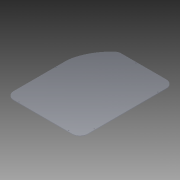
# Autodesk Inventor part: metacrilat proteccio dret
Saved by Autodesk Inventor 2012 SP1 (Build 160190100, 190)
## iProperties
Created: 2015-03-29
Part Number: metacrilat proteccio dret
Material: Default
Document SubType Name: Modeling
Designer: sheina
Density: 1 g/cm^3
Author: sheina
Autodesk Inventor part; units mm, degrees
ref_plane "YZ Plane" through (0, 0, 0) normal (1, 0, 0) x (0, 1, 0)
ref_plane "XZ Plane" through (0, 0, 0) normal (0, 1, 0) x (-1, 0, 0)
ref_plane "XY Plane" through (0, 0, 0) normal (0, 0, 1) x (1, 0, 0)
sketch "Boceto1" plane through (0, 0, 0) normal (0, 0, 1) x (1, 0, 0)
  line L0 (200.6138, -49.1011) -> (347.0892, -49.1011)
  line L1 (366.6054, -71.1) -> (366.6054, -332.1)
  line L2 (352.0892, -357.1011) -> (151.6064, -357.1011)
  line L3 (124.6054, -332.1) -> (124.6054, -152.9933)
  line L4 (366.6054, -332.1) -> (366.6054, -357.1011)
  line L5 (352.0892, -357.1011) -> (366.6054, -357.1011)
  line L6 (347.0892, -49.1011) -> (366.6054, -49.1011)
  line L7 (366.6054, -71.1) -> (366.6054, -49.1011)
  line L8 (151.6064, -357.1011) -> (124.6054, -357.1011)
  line L9 (124.6054, -332.1) -> (124.6054, -357.1011)
  line L10 (200.6138, -49.1011) -> (185.295, -49.1011)
  arc A0 (185.295, -49.1011) -> (124.6054, -152.9933) centre (292.3571, -181.3147) ccw
  dimension "d2" = 308
  dimension "d3" = 242
  constraints: 22 end point, 5 perpendicular, 2 parallel, 2 point on circle, 1 centre point
  measures "d2" distance between parallel lines of L2 L0
  measures "d3" distance between parallel lines of L3 L1
extrude "Extrusión2" add sketch "Boceto1" along normal blind 2
fillet "Empalme1" radius 25 3 edges at (366.6054, -49.1011, 1) (366.6054, -357.1011, 1) (124.6054, -357.1011, 1)
sketch "Boceto3" plane through (0, 0, 2) normal (0, 0, 1) x (1, 0, 0)
  line L0 (341.6054, -357.1011) -> (149.6054, -357.1011) projected
  line L1 (366.6054, -74.1011) -> (366.6054, -332.1011) projected
  line L2 (185.295, -49.1011) -> (341.6054, -49.1011) projected
  line L3 (124.6054, -332.1011) -> (124.6054, -152.9933) projected
  circle A0 centre (164.6054, -354.1011) radius 1.75
  circle A1 centre (326.6054, -354.1011) radius 1.75
  circle A2 centre (127.6054, -196.1011) radius 1.75
  circle A3 centre (363.6054, -307.1011) radius 1.75
  circle A4 centre (363.6054, -99.1011) radius 1.75
  circle A5 centre (245.1054, -52.1011) radius 1.75
  point P0 (200.6138, -49.1011)
  point P1 (0, 0)
  dimension "d7" = 3.5
  dimension "d8" = 3.5
  dimension "d9" = 3.5
  dimension "d10" = 3.5
  dimension "d11" = 3.5
  dimension "d12" = 3.5
  dimension "d13" = 3
  dimension "d14" = 3
  dimension "d15" = 3
  dimension "d16" = 3
  dimension "d17" = 3
  dimension "d18" = 3
  dimension "d19" = 121.5
  dimension "d20" = 161
  dimension "d21" = 50
  dimension "d22" = 50
  dimension "d23" = 40
  dimension "d24" = 40
  constraints: 6 centre point
  measures "d7" diameter of A0
  measures "d8" diameter of A1
  measures "d9" diameter of A2
  measures "d10" diameter of A3
  measures "d11" diameter of A4
  measures "d12" diameter of A5
  measures "d13" distance from line of L3 A2.centre
  measures "d14" distance from line of L0 A0.centre
  measures "d15" distance from line of L0 A1.centre
  measures "d16" distance from line of L1 A3.centre
  measures "d17" distance from line of L1 A4.centre
  measures "d18" distance from line of L2 A5.centre
  measures "d19" distance from line of A5.centre L1
  measures "d20" distance from line of A2.centre L0
  measures "d21" distance from line of L0 A3.centre
  measures "d22" distance from line of A4.centre L2
  measures "d23" distance from line of A0.centre L3
  measures "d24" horizontal distance of L1.end A1.centre
extrude "Extrusión3" cut sketch "Boceto3" against normal blind 2
fillet "Empalme2" radius 20 1 edges at (185.295, -49.1011, 1)
fillet "Empalme3" radius 100 1 edges at (124.6054, -152.9933, 1)
equation "\"d14\" = d13"
equation "\"d15\" = d13"
equation "\"d16\" = d13"
equation "\"d17\" = d13"
equation "\"d18\" = d13"
